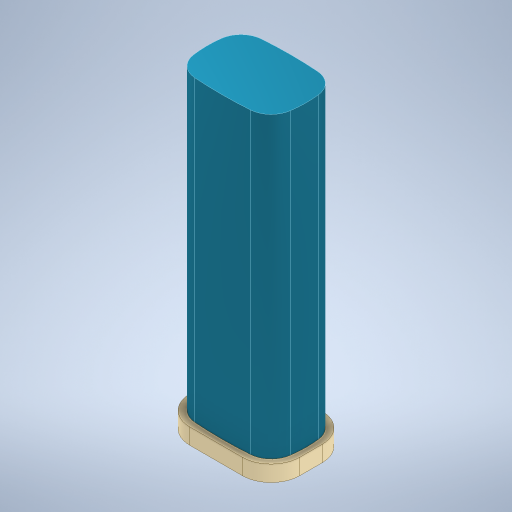
# Autodesk Inventor part: vape-tube-test-print
Saved by Autodesk Inventor 2023 (Build 270158030, 158C)
## iProperties
Created: 2023-11-17
Part Number: vape-tube-test-print
Material: Generic
Document SubType Name: Modeling
Designer: Imogen Heard
Density: 1 g/cm^3
Appearance: Anodized blue
Author: Imogen Heard
Autodesk Inventor part; units mm, degrees
ref_plane "YZ Plane" through (0, 0, 0) normal (1, 0, 0) x (0, 1, 0)
ref_plane "XZ Plane" through (0, 0, 0) normal (0, 1, 0) x (-1, 0, 0)
ref_plane "XY Plane" through (0, 0, 0) normal (0, 0, 1) x (1, 0, 0)
sketch "Sketch1" plane through (0, 0, 0) normal (0, 1, 0) x (-1, 0, 0)
  line L0 (15.5, -10.8) -> (-15.5, -10.8) construction
  line L1 (-15.5, -10.8) -> (-15.5, 10.8) construction
  line L2 (-15.5, 10.8) -> (15.5, 10.8) construction
  line L3 (15.5, 10.8) -> (15.5, -10.8) construction
  line L4 (15.5, -9.8) -> (0, -11.8) construction
  line L5 (0, -11.8) -> (-15.5, -9.8) construction
  spline S0 degree 2 poles (15.5, -9.8) (0, -11.8) (-15.5, -9.8) knots 1 1 1 2 2 2
  line L6 (15.5, 9.8) -> (0, 11.8) construction
  line L7 (0, 11.8) -> (-15.5, 9.8) construction
  spline S1 degree 2 poles (15.5, 9.8) (0, 11.8) (-15.5, 9.8) knots 1 1 1 2 2 2
  line L8 (-15.5, -9.8) -> (-15.5, 9.8)
  line L9 (15.5, 9.8) -> (15.5, -9.8)
  line L10 (13.5, -10.8) -> (13.3899, -12.4573) construction
  line L11 (13.3858, 11.8689) -> (13.5, 10.8) construction
  spline S2 degree 2 poles (13.95, 9.99) (13.3858, 11.8689) (13.5, 10.8) knots 0 0 0 1 1 1 construction
  spline S3 degree 2 poles (13.5, -10.8) (13.3899, -12.4573) (14.1, -9.9725) knots 0 0 0 1 1 1 construction
  line L12 (13.3899, -12.4573) -> (14.1, -9.9725) construction
  line L13 (14.1, -9.9725) -> (16.95, 0) construction
  spline S4 degree 2 poles (14.1, -9.9725) (16.95, 0) (13.95, 9.99) knots 1.076223 1.076223 1.076223 1.923777 1.923777 1.923777
  line L14 (16.95, 0) -> (13.95, 9.99) construction
  line L15 (13.95, 9.99) -> (13.3858, 11.8689) construction
  line L16 (0, 3.4411) -> (0, -4.0542)
  line L17 (-14.1, -9.9725) -> (-16.95, 0) construction
  spline S5 degree 2 poles (-14.1, -9.9725) (-16.95, 0) (-13.95, 9.99) knots 1.076223 1.076223 1.076223 1.923777 1.923777 1.923777
  line L18 (-16.95, 0) -> (-13.95, 9.99) construction
  point P0 (0, 0)
  point P1 (-15.977, 0)
  point P2 (-15.977, 0)
  point P3 (15.5, 0)
  point P4 (-15.5, 0)
  point P5 (15.5, 0)
  point P6 (-15.5, -1.3514)
  point P7 (-14.1, -9.9725)
  point P8 (15.5, -1.3514)
  point P9 (15.5, 1.0529)
  point P10 (-13.95, 9.99)
  point P11 (-15.5, 1.0529)
  dimension "d0" = 31
  dimension "d1" = 15.5
  dimension "d2" = 21.6
  dimension "d3" = 10.8
  dimension "d6" = 1
  dimension "d7" = 15.5
  dimension "d8" = 2
  dimension "d10" = 2
  dimension "d13" = 1.55
  dimension "d14" = 1.4
  dimension "d15" = 3
  constraints: 14 end point, 5 vertical alignment, 4 horizontal alignment, 4 point on line, 3 midpoint, 3 parallel, 3 symmetric about line, 2 vertical, 1 coincident, 1 horizontal, 1 perpendicular, 21 other
  measures "d0" distance between parallel lines of L1 L3
  measures "d1" distance from line of point (0, 0) L3
  measures "d2" distance between parallel lines of L2 L0
  measures "d3" distance from line of point (0, 0) L0
  measures "d6" distance from line of L0 L4.start
  measures "d7" distance from line of L3 L4.end
  measures "d8" vertical distance of L4.start L4.end
  measures "d10" distance from line of L10.start L3
  measures "d13" horizontal distance of point (15.5, 0) L14.end
  measures "d14" horizontal distance of point (15.5, 0) L12.end
  measures "d15" horizontal distance of L14.end L13.end
extrude "Extrusion1" add sketch "Sketch1" along normal blind 98.5 contours S0 S5 S1 S4
fillet "Fillet1" radius 7 4 edges at (13.95, 49.25, 9.99) (-13.95, 49.25, 9.99) (14.1, 49.25, -9.9725) (-14.1, 49.25, -9.9725)
sketch "Sketch2" plane through (0, 0, 0) normal (0, -1, 0) x (1, 0, 0)
  spline S0 degree 6 poles (-8.8058, -10.4772) (-9.1759, -10.4501) (-9.5527, -10.3988) (-9.9335, -10.3215) (-10.3153, -10.2169) (-10.6942, -10.0841) (-11.4392, -9.7628) (-11.8052, -9.5742) (-12.1608, -9.3579) (-12.5022, -9.1149) (-12.8258, -8.8475) (-13.4314, -8.2691) (-13.7134, -7.9582) (-13.9718, -7.6284) (-14.2043, -7.283) (-14.4095, -6.9261) (-14.7648, -6.1967) (-14.9148, -5.8243) (-15.037, -5.4478) (-15.1317, -5.0709) (-15.2002, -4.6969) (-15.2444, -4.3284) knots 0 0 0 0 0 0 0 0.249928 0.249928 0.249928 0.249928 0.249928 0.5 0.5 0.5 0.5 0.5 0.750072 0.750072 0.750072 0.750072 0.750072 1 1 1 1 1 1 1 projected
  spline S1 degree 2 poles (8.8058, -10.4772) (0, -11.1228) (-8.8058, -10.4772) knots 0 0 0 1 1 1 projected
  spline S2 degree 6 poles (15.2444, -4.3284) (15.2002, -4.6969) (15.1317, -5.0709) (15.037, -5.4478) (14.9148, -5.8243) (14.7648, -6.1967) (14.4095, -6.9261) (14.2043, -7.283) (13.9718, -7.6284) (13.7134, -7.9582) (13.4314, -8.2691) (12.8258, -8.8475) (12.5022, -9.1149) (12.1608, -9.3579) (11.8052, -9.5742) (11.4392, -9.7628) (10.6942, -10.0841) (10.3153, -10.2169) (9.9335, -10.3215) (9.5527, -10.3988) (9.1759, -10.4501) (8.8058, -10.4772) knots 0 0 0 0 0 0 0 0.249928 0.249928 0.249928 0.249928 0.249928 0.5 0.5 0.5 0.5 0.5 0.750072 0.750072 0.750072 0.750072 0.750072 1 1 1 1 1 1 1 projected
  spline S3 degree 2 poles (15.1628, 4.4592) (15.7704, 0.0637) (15.2444, -4.3284) knots 0 0 0 1 1 1 projected
  spline S4 degree 6 poles (8.7365, 10.4823) (9.1027, 10.4557) (9.4753, 10.4054) (9.8517, 10.3298) (10.229, 10.2274) (10.6036, 10.0977) (11.3404, 9.7839) (11.7025, 9.5998) (12.0547, 9.3886) (12.3931, 9.1516) (12.7144, 8.8905) (13.3169, 8.3258) (13.5982, 8.0221) (13.8567, 7.6997) (14.0902, 7.3619) (14.2974, 7.0125) (14.6582, 6.2976) (14.8119, 5.9321) (14.9384, 5.5623) (15.0383, 5.1915) (15.1125, 4.8229) (15.1628, 4.4592) knots 0 0 0 0 0 0 0 0.249931 0.249931 0.249931 0.249931 0.249931 0.5 0.5 0.5 0.5 0.5 0.750069 0.750069 0.750069 0.750069 0.750069 1 1 1 1 1 1 1 projected
  spline S5 degree 2 poles (-8.7365, 10.4823) (0, 11.1177) (8.7365, 10.4823) knots 0 0 0 1 1 1 projected
  spline S6 degree 6 poles (-15.1628, 4.4592) (-15.1125, 4.8229) (-15.0383, 5.1915) (-14.9384, 5.5623) (-14.8119, 5.9321) (-14.6582, 6.2976) (-14.2974, 7.0125) (-14.0902, 7.3619) (-13.8567, 7.6997) (-13.5982, 8.0221) (-13.3169, 8.3258) (-12.7144, 8.8905) (-12.3931, 9.1516) (-12.0547, 9.3886) (-11.7025, 9.5998) (-11.3404, 9.7839) (-10.6036, 10.0977) (-10.229, 10.2274) (-9.8517, 10.3298) (-9.4753, 10.4054) (-9.1027, 10.4557) (-8.7365, 10.4823) knots 0 0 0 0 0 0 0 0.249931 0.249931 0.249931 0.249931 0.249931 0.5 0.5 0.5 0.5 0.5 0.750069 0.750069 0.750069 0.750069 0.750069 1 1 1 1 1 1 1 projected
  spline S7 degree 2 poles (-15.2444, -4.3284) (-15.7704, 0.0637) (-15.1628, 4.4592) knots 0 0 0 1 1 1 projected
  line L0 (-8.2444, 12.4823) -> (8.1628, 12.4823)
  line L1 (17.1628, 3.4823) -> (17.1628, -3.4772)
  line L2 (8.1628, -12.4772) -> (-8.2444, -12.4772)
  line L3 (-17.2444, -3.4772) -> (-17.2444, 3.4823)
  arc A0 (-8.2444, 12.4823) -> (-17.2444, 3.4823) centre (-8.2444, 3.4823) ccw
  arc A1 (17.1628, 3.4823) -> (8.1628, 12.4823) centre (8.1628, 3.4823) ccw
  arc A2 (8.1628, -12.4772) -> (17.1628, -3.4772) centre (8.1628, -3.4772) ccw
  arc A3 (-17.2444, -3.4772) -> (-8.2444, -12.4772) centre (-8.2444, -3.4772) ccw
  point P0 (0, 0)
  dimension "d17" = 2
  dimension "d18" = 2
  dimension "d19" = 2
  dimension "d20" = 2
  dimension "d21" = 9
  constraints: 8 end point, 8 point on circle, 8 tangent, 4 centre point, 3 equal radius, 2 horizontal alignment, 2 parallel, 1 horizontal, 1 perpendicular, 6 other
  measures "d17" distance from line of L0 point (-8.737, 10.482)
  measures "d18" distance from line of L3 point (-15.244, -4.328)
  measures "d19" distance from line of L2 point (-8.806, -10.477)
  measures "d20" distance from line of L1 point (15.163, 4.459)
  measures "d21" radius of A0
extrude "Extrusion2" add sketch "Sketch2" against normal blind 5 separate body
equation "\"d1\" = 0.5 * d0"
equation "\"d3\" = 0.5 * d2"
equation "\"d7\" = d1"
equation "\"d19\" = d18"
equation "\"d20\" = d18"
